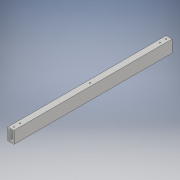
# Autodesk Inventor part: 26in 2x1
Saved by Autodesk Inventor 2018 (Build 220112000, 112)
## iProperties
Created: 2018-12-20
Part Number: 26in 2x1
Material: Generic
Document SubType Name: Modeling
Designer: maste
Density: 1 g/cm^3
Appearance: Default
Author: maste
Autodesk Inventor part; units mm, degrees
ref_plane "YZ Plane" through (0, 0, 0) normal (1, 0, 0) x (0, 1, 0)
ref_plane "XZ Plane" through (0, 0, 0) normal (0, 1, 0) x (-1, 0, 0)
ref_plane "XY Plane" through (0, 0, 0) normal (0, 0, 1) x (1, 0, 0)
sketch "Sketch1" plane through (0, 0, 0) normal (0, 0, 1) x (1, 0, 0)
  line L0 (0, 0) -> (25.4, 0)
  line L1 (25.4, 0) -> (25.4, 50.8)
  line L2 (25.4, 50.8) -> (0, 50.8)
  line L3 (0, 50.8) -> (0, 0)
  line L4 (21.59, 46.99) -> (21.59, 3.81)
  line L5 (21.59, 3.81) -> (3.81, 3.81)
  line L6 (3.81, 3.81) -> (3.81, 46.99)
  line L7 (3.81, 46.99) -> (21.59, 46.99)
  dimension "d0" = 25.4
  dimension "d1" = 50.8
  dimension "d2" = 3.81
  constraints: 16 end point, 4 parallel, 2 perpendicular, 1 horizontal, 3 other
  measures "d0" distance of L2.end L1.end
  measures "d1" distance of L1.end L0.end
  measures "d2" distance between parallel lines of L1 L4
extrude "Extrusion1" add sketch "Sketch1" along normal blind 660.4
sketch "Sketch2" plane through (0, 50.8, 0) normal (0, 1, 0) x (1, 0, 0)
  line L0 (0, 0) -> (25.4, 0) projected
  line L1 (12.7, 0) -> (12.7, -660.4) construction
  line L2 (0, -660.4) -> (25.4, -660.4) projected
  line L3 (12.7, 0) -> (12.7, -12.7) construction
  line L4 (12.7, -12.7) -> (12.7, -38.1) construction
  line L5 (12.7, -660.4) -> (12.7, -647.7) construction
  line L6 (12.7, -647.7) -> (12.7, -622.3) construction
  line L7 (0, 0) -> (0, -660.4) construction
  line L8 (0, -330.2) -> (25.4, -330.2) construction
  circle A0 centre (12.7, -647.7) radius 2.54
  circle A1 centre (12.7, -622.3) radius 2.54
  circle A2 centre (12.7, -330.2) radius 2.54
  circle A3 centre (12.7, -38.1) radius 2.54
  circle A4 centre (12.7, -12.7) radius 2.54
  dimension "d5" = 12.7
  dimension "d6" = 25.4
  dimension "d7" = 12.7
  dimension "d8" = 25.4
  dimension "d9" = 5.08
  constraints: 12 end point, 5 centre point, 4 coincident, 4 midpoint, 4 point on line, 1 horizontal
  measures "d5" distance of L1.start L3.end
  measures "d6" distance of L3.end L4.end
  measures "d7" distance of L1.end L5.end
  measures "d8" distance of L5.end L6.end
  measures "d9" diameter of A0
extrude "Extrusion2" cut sketch "Sketch2" against normal blind 660.4
body "Solid1"
